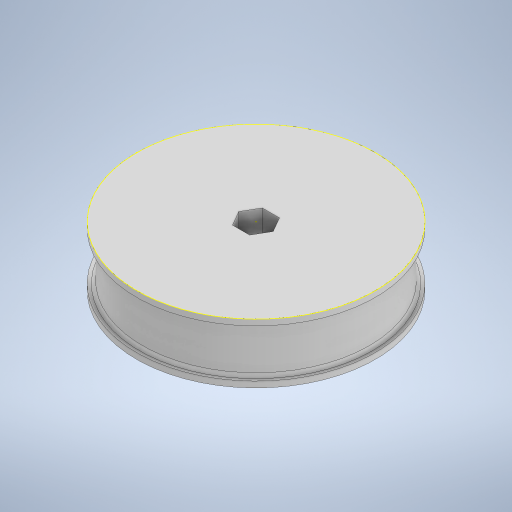
# Autodesk Inventor part: 4-bar intake () pully
Saved by Autodesk Inventor 2023 (Build 270158030, 158C)
## iProperties
Created: 2022-07-18
Part Number: 4-bar intake () pully
Material: Generic
Document SubType Name: Modeling
Designer: kt1040502
Density: 1 g/cm^3
Appearance: Default
Author: kt1040502
Autodesk Inventor part; units mm, degrees
ref_plane "YZ Plane" through (0, 0, 0) normal (1, 0, 0) x (0, 1, 0)
ref_plane "XZ Plane" through (0, 0, 0) normal (0, 1, 0) x (-1, 0, 0)
ref_plane "XY Plane" through (0, 0, 0) normal (0, 0, 1) x (1, 0, 0)
sketch "Sketch1" plane through (0, 0, 0) normal (0, 0, 1) x (1, 0, 0)
  line L0 (0, 0) -> (50.8, 0)
  line L1 (50.8, 0) -> (50.8, 25.4)
  line L2 (50.8, 25.4) -> (0, 25.4)
  line L3 (0, 25.4) -> (0, 0)
  line L4 (0, 22.86) -> (1.27, 22.86)
  line L5 (2.54, 21.59) -> (2.54, 3.81)
  line L6 (1.27, 2.54) -> (0, 2.54)
  arc A0 (2.54, 21.59) -> (1.27, 22.86) centre (1.27, 21.59) ccw
  arc A1 (1.27, 2.54) -> (2.54, 3.81) centre (1.27, 3.81) ccw
  point P0 (0.635, 22.86)
  point P1 (0.635, 2.54)
  point P2 (41.91, 0)
  point P3 (41.91, 25.4)
  dimension "d0" = 50.8
  dimension "d1" = 25.4
  dimension "d2" = 2.54
  dimension "d3" = 2.54
  dimension "d4" = 2.54
  dimension "d5" = 1.27
  constraints: 14 end point, 4 point on circle, 4 point on line, 4 tangent, 3 perpendicular, 2 centre point, 2 horizontal, 2 midpoint, 2 parallel, 1 equal radius
  measures "d0" distance of L2.end L1.end
  measures "d1" distance of L1.end L0.end
  measures "d2" distance from line of L2 point (0.635, 22.86)
  measures "d3" distance from line of L0 point (0.635, 2.54)
  measures "d4" distance between parallel lines of L5 L3
  measures "d5" radius of A0
revolve "Revolution1" add sketch "Sketch1" angle 360 about axis through (50.8, 0, 0) along (0, 1, 0) contours L3 L6 A1 L5 A0 L4 L2 L1 L0
sketch "Sketch2" plane through (50.8, 25.4, 0) normal (0, 1, 0) x (1, 0, 0)
  circle A0 centre (0, 0) radius 50.8 projected
  point P0 (-50.8, 0)
  constraints: 1 horizontal alignment
sketch "Sketch3" plane through (50.8, 25.4, 0) normal (0, 1, 0) x (1, 0, 0)
  circle A0 centre (0, 0) radius 6.35
  circle A1 centre (0, 0) radius 50.8 projected
  line L0 (3.6662, 6.35) -> (7.3323, 0)
  line L1 (7.3323, 0) -> (3.6662, -6.35)
  line L2 (3.6662, -6.35) -> (-3.6662, -6.35)
  line L3 (-3.6662, -6.35) -> (-7.3323, 0)
  line L4 (-7.3323, 0) -> (-3.6662, 6.35)
  line L5 (-3.6662, 6.35) -> (3.6662, 6.35)
  point P0 (-50.8, 0)
  point P1 (0, 6.35)
  dimension "d9" = 12.7
  constraints: 12 end point, 1 coincident, 1 horizontal alignment, 1 midpoint, 1 vertical alignment, 15 other
extrude "Extrusion1" cut sketch "Sketch3" against normal blind 25.4 contours A0 | A0 L0 L1 | A0 L5 L0 | L1 L2 A0 | A0 L4 L5 | L2 L3 A0 | A0 L3 L4
body "Solid1"
